qcxrfgain (Autodesk Fusion 360 design; units mm, degrees)
Autodesk Fusion 360 part; units mm, degrees
sketch "Sketch1" plane through (0, 0, 0) normal (0, 0, 1) x (1, 0, 0)
  circle A0 centre (0, 0) radius 3
  circle A1 centre (0, 0) radius 5
  dimension "d1" = 6
  dimension "d4" = 10
  constraint coincident A0.centre A1.centre
  constraint concentric A0 A1
  measures "d1" diameter of A0
  measures "d4" diameter of A1
extrude "Extrude1" add sketch "Sketch1" along normal blind 11 contours A0
extrude "Extrude2" add sketch "Sketch1" against normal blind 13 contours A0 | A1
ref_plane "WorkPlane1" through (0, 0, -15) normal (0, 0, 1) x (1, 0, 0)
sketch "Sketch2" plane through (0, 0, -15) normal (0, 0, 1) x (1, 0, 0)
  circle A0 centre (0, 0) radius 3.25
  dimension "d8" = 6.5
  constraint coincident A0.centre origin
  measures "d8" diameter of A0
extrude "Extrude3" cut sketch "Sketch2" along normal blind 11
